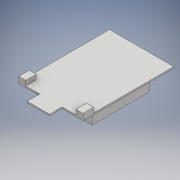
# Autodesk Inventor part: terminal
Saved by Autodesk Inventor 2017.3 (Build 213256000, 256)
## iProperties
Part Number: terminal
Material: 一般
Document SubType Name: Modeling
Designer: sktom
Density: 1 g/cm^3
Appearance: 既定
Author: sktom
Autodesk Inventor part; units mm, degrees
ref_plane "YZ Plane" through (0, 0, 0) normal (1, 0, 0) x (0, 1, 0)
ref_plane "XZ Plane" through (0, 0, 0) normal (0, 1, 0) x (-1, 0, 0)
ref_plane "XY Plane" through (0, 0, 0) normal (0, 0, 1) x (1, 0, 0)
sketch "スケッチ1" plane through (0, 0, 0) normal (0, 0, 1) x (1, 0, 0)
  line L0 (-4.6, -6.5) -> (4.6, -6.5)
  line L1 (4.6, -6.5) -> (4.6, 6.5)
  line L2 (4.6, 6.5) -> (-4.6, 6.5)
  line L3 (-4.6, 6.5) -> (-4.6, -6.5)
  line L4 (-4.6, -6.5) -> (4.6, 6.5) construction
  line L5 (4.6, -6.5) -> (-4.6, 6.5) construction
  point P0 (0, 0)
  dimension "d0" = 9.2
  dimension "d1" = 13
  constraints: 12 end point, 2 midpoint, 2 parallel, 1 horizontal, 1 perpendicular
  measures "d0" distance of L2.end L1.end
  measures "d1" distance of L0.end L1.end
extrude "押し出し1" add sketch "スケッチ1" along normal blind 0.2
sketch "スケッチ2" plane through (0, 0, 0.2) normal (0, 0, 1) x (1, 0, 0)
  line L0 (-4.6, -6.5) -> (-3.6, -6.5)
  line L1 (-3.6, -6.5) -> (-3.6, -5)
  line L2 (-3.6, -5) -> (-4.6, -5)
  line L3 (-4.6, -5) -> (-4.6, -6.5)
  line L4 (-4.6, -6.5) -> (4.6, -6.5) projected
  line L5 (4.6, -6.5) -> (3.6, -6.5)
  line L6 (3.6, -6.5) -> (3.6, -5)
  line L7 (3.6, -5) -> (4.6, -5)
  line L8 (4.6, -5) -> (4.6, -6.5)
  point P0 (0, 0)
  dimension "d4" = 1.5
  dimension "d5" = 1
  constraints: 16 end point, 4 parallel, 2 coincident, 2 equal length, 2 horizontal, 2 perpendicular
  measures "d4" distance of L0.end L1.end
  measures "d5" distance of L1.end L2.end
extrude "押し出し2" add sketch "スケッチ2" along normal blind 0.7
sketch "スケッチ3" plane through (0, 0, 0) normal (0, 0, -1) x (-1, 0, 0)
  line L0 (-2.3, -2.9) -> (2.3, -2.9)
  line L1 (2.3, -2.9) -> (2.3, 5.3)
  line L2 (2.3, 5.3) -> (-2.3, 5.3)
  line L3 (-2.3, 5.3) -> (-2.3, -2.9)
  line L4 (-2.3, -2.9) -> (2.3, 5.3) construction
  line L5 (2.3, -2.9) -> (-2.3, 5.3) construction
  line L6 (-4.6, 6.5) -> (4.6, 6.5) projected
  point P0 (0, 0)
  point P1 (0, 1.2)
  point P2 (0, 1.2)
  dimension "d8" = 1.2
  dimension "d9" = 4.6
  dimension "d10" = 8.2
  constraints: 12 end point, 3 midpoint, 2 parallel, 1 horizontal, 1 perpendicular, 1 vertical alignment
  measures "d8" distance between parallel lines of L6 L2
  measures "d9" distance of L1.end L2.end
  measures "d10" distance of L0.end L1.end
extrude "押し出し3" add sketch "スケッチ3" along normal blind 3.5
sketch "スケッチ4" plane through (0, 0, 0) normal (0, 0, -1) x (-1, 0, 0)
  line L0 (-1.6, -6.5) -> (1.6, -6.5)
  line L1 (1.6, -6.5) -> (1.6, -8.3)
  line L2 (1.6, -8.3) -> (-1.6, -8.3)
  line L3 (-1.6, -8.3) -> (-1.6, -6.5)
  line L4 (4.6, -6.5) -> (-4.6, -6.5) projected
  point P0 (0, 0)
  point P1 (0, -6.5)
  point P2 (0, -6.5)
  dimension "d13" = 3.2
  dimension "d14" = 1.8
  constraints: 8 end point, 2 midpoint, 2 parallel, 1 coincident, 1 horizontal, 1 horizontal alignment, 1 perpendicular
  measures "d13" distance of L0.start L0.end
  measures "d14" distance of L0.end L1.end
extrude "押し出し4" add sketch "スケッチ4" against normal up to surface (0.2 mm away)
